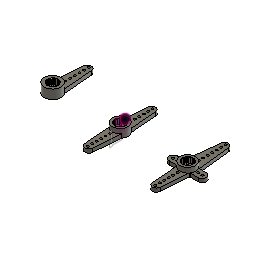
MG90_Arm (Autodesk Fusion 360 design; units mm, degrees)
Autodesk Fusion 360 part; units mm, degrees
sketch "Arm01Base" plane through (0, 0, 0) normal (0, 1, 0) x (1, 0, 0)
  circle A0 centre (0, 0) radius 3.7
  circle A1 centre (0, 0) radius 2.7
  line L0 (0, -3.7) -> (0, 17.2) construction
  circle A2 centre (0, 15.45) radius 1.75
  line L1 (-1.7434, 15.6016) -> (-2.9, 2.2978)
  line L2 (1.7434, 15.6016) -> (2.9, 2.2978)
  circle A3 centre (0, 0) radius 1.375
  circle A4 centre (0, 16.05) radius 0.5
  circle A5 centre (0, 13.98) radius 0.5
  circle A6 centre (0, 11.91) radius 0.5
  circle A7 centre (0, 9.84) radius 0.5
  circle A8 centre (0, 7.77) radius 0.5
  circle A9 centre (0, 5.7) radius 0.5
  point P0 (0, 16.55)
  dimension "d2" = 7.4
  dimension "d3" = 1
  dimension "d4" = 20.9
  dimension "d5" = 3.5
  dimension "d6" = 2.9
  dimension "d7" = 2.75
  dimension "d8" = 1
  dimension "d9" = 0.65
  dimension "d12" = 0
  dimension "d13" = -10.35
  constraint coincident A0.centre A1.centre
  constraint coincident A0 L0.start
  constraint vertical L0
  constraint coincident A0.centre L0
  constraint coincident L0 A2.centre
  constraint coincident L0.end A2
  constraint coincident A2 L1.start
  constraint coincident A0 L1.end
  constraint tangent A2 L1
  constraint symmetric L0 L1.start L2.start
  constraint symmetric L0 L1.end L2.end
  constraint concentric A1 A3
  constraint coincident L0 A4.centre
  constraint coincident A4 P0
  constraint coincident L0 P0
  measures "d2" diameter of A0
  measures "d3" distance of A0 A1
  measures "d4" distance of L0.start L0.end
  measures "d5" diameter of A2
  measures "d6" distance of L0 L1.end
  measures "d7" diameter of A3
  measures "d8" diameter of A4
  measures "d9" distance of L0.end P0
extrude "Extrude1" add sketch "Arm01Base" along normal blind 1.75 contours A0 | A0 A2 L1 L2 A5 | A2 A5 picked at (0.7406, 14.9094) makes body 1
extrude "Extrude2" add sketch "Arm01Base" along normal blind 4.1 contours A0 bodies 1
ref_plane "WorkPlane1" through (0, 1.5, 0) normal (0, 1, 0) x (0, 0, 1)
extrude "Extrude3" add sketch "Arm01Base" against normal blind 0.5 from surface at 1.5 contours A1 bodies 1
sketch "Teeth01" plane through (0, 1.5, 0) normal (0, 1, 0) x (1, 0, 0)
  circle A0 centre (0, 0) radius 2.1 construction
  circle A1 centre (0, 0) radius 2.4 construction
  line L0 (0, 0) -> (0, 2.4) construction
  line L1 (-0.35, 2.3743) -> (0, 2.1)
  line L2 (0.35, 2.3743) -> (0, 2.1)
  line L3 (-1.0666, 2.15) -> (-0.6489, 1.9972)
  line L4 (-0.4008, 2.3663) -> (-0.6489, 1.9972)
  line L5 (-1.6788, 1.7152) -> (-1.2343, 1.6989)
  line L6 (-1.1124, 2.1266) -> (-1.2343, 1.6989)
  line L7 (-2.1266, 1.1124) -> (-1.6989, 1.2343)
  line L8 (-1.7152, 1.6788) -> (-1.6989, 1.2343)
  line L9 (-2.3663, 0.4008) -> (-1.9972, 0.6489)
  line L10 (-2.15, 1.0666) -> (-1.9972, 0.6489)
  line L11 (-2.3743, -0.35) -> (-2.1, 0)
  line L12 (-2.3743, 0.35) -> (-2.1, 0)
  line L13 (-2.15, -1.0666) -> (-1.9972, -0.6489)
  line L14 (-2.3663, -0.4008) -> (-1.9972, -0.6489)
  line L15 (-1.7152, -1.6788) -> (-1.6989, -1.2343)
  line L16 (-2.1266, -1.1124) -> (-1.6989, -1.2343)
  line L17 (-1.1124, -2.1266) -> (-1.2343, -1.6989)
  line L18 (-1.6788, -1.7152) -> (-1.2343, -1.6989)
  line L19 (-0.4008, -2.3663) -> (-0.6489, -1.9972)
  line L20 (-1.0666, -2.15) -> (-0.6489, -1.9972)
  line L21 (0.35, -2.3743) -> (0, -2.1)
  line L22 (-0.35, -2.3743) -> (0, -2.1)
  line L23 (1.0666, -2.15) -> (0.6489, -1.9972)
  line L24 (0.4008, -2.3663) -> (0.6489, -1.9972)
  line L25 (1.6788, -1.7152) -> (1.2343, -1.6989)
  line L26 (1.1124, -2.1266) -> (1.2343, -1.6989)
  line L27 (2.1266, -1.1124) -> (1.6989, -1.2343)
  line L28 (1.7152, -1.6788) -> (1.6989, -1.2343)
  line L29 (2.3663, -0.4008) -> (1.9972, -0.6489)
  line L30 (2.15, -1.0666) -> (1.9972, -0.6489)
  line L31 (2.3743, 0.35) -> (2.1, 0)
  line L32 (2.3743, -0.35) -> (2.1, 0)
  line L33 (2.15, 1.0666) -> (1.9972, 0.6489)
  line L34 (2.3663, 0.4008) -> (1.9972, 0.6489)
  line L35 (1.7152, 1.6788) -> (1.6989, 1.2343)
  line L36 (2.1266, 1.1124) -> (1.6989, 1.2343)
  line L37 (1.1124, 2.1266) -> (1.2343, 1.6989)
  line L38 (1.6788, 1.7152) -> (1.2343, 1.6989)
  line L39 (0.4008, 2.3663) -> (0.6489, 1.9972)
  line L40 (1.0666, 2.15) -> (0.6489, 1.9972)
  circle A2 centre (0, 0) radius 2.7
  circle A3 centre (0, 0) radius 2.4
  dimension "d22" = 4.2
  dimension "d23" = 4.8
  dimension "d24" = 0.35
  dimension "d26" = 360
  constraint coincident A0.centre A1.centre
  constraint concentric A0 A1
  constraint coincident A1 L0.end
  constraint vertical L0
  constraint coincident A1 L1.start
  constraint coincident A0 L1.end
  constraint coincident L0 L1.end
  constraint coincident A1 L2.start
  constraint symmetric L0 L1.start L2.start
  constraint coincident L39.start A3
  measures "d22" diameter of A0
  measures "d23" diameter of A1
  measures "d24" horizontal distance of L0.end L2.start
extrude "Extrude4" add sketch "Teeth01" along normal up to surface (2.6 mm away) contours L1 L2 A3 | L3 L4 A3 | L39 L40 A3 | L5 L6 A3 | L37 L38 A3 | L7 L8 A3 | L35 L36 A3 | L9 L10 A3 | L33 L34 A3 | L11 L12 A3 | L31 L32 A3 | L13 L14 A3 | L29 L30 A3 | L15 L16 A3 | L27 L28 A3 | L17 L18 A3 | L25 L26 A3 | L19 L20 A3 | L23 L24 A3 | L21 L22 A3 | A2 bodies 1
sketch "TeethChamfer01" plane through (0, 0, 0) normal (1, 0, 0) x (0, 0, -1)
  line L0 (3.7, 4.1) -> (-3.7, 4.1) construction
  line L1 (0, 0) -> (0, 4.1) construction
  line L2 (2.3743, 4.1) -> (2.1, 3.8)
  line L3 (2.1, 3.8) -> (2.1, 4.1)
  line L4 (2.3743, 4.1) -> (2.1, 4.1)
  point P0 (2.3743, 4.1)
  point P1 (2.1, 4.1)
  dimension "d29" = 0.3
  constraint coincident L1.start origin
  constraint midpoint L0 L1.end
  constraint coincident P0 L2.start
  constraint coincident L0 P1
  constraint perpendicular L0 L3
  constraint coincident P1 L3.end
  measures "d29" distance of L2.end P1
revolve "Revolve1" cut sketch "TeethChamfer01" angle 360 about axis through (0, 0, 0) along (0, 1, 0) bodies 1
copy_body "Body->Comp1" bodies 1 removing the originals makes body 2 in component "Arm01"
sketch "Arm02Base" plane through (0, 0, 0) normal (0, 1, 0) x (1, 0, 0)
  line L0 (0, 0) -> (30, 0) construction
  circle A0 centre (30, 0) radius 3.45
  circle A1 centre (30, 0) radius 2.25
  line L1 (30, -15.675) -> (30, 15.675) construction
  circle A2 centre (30, 13.925) radius 1.75
  line L2 (28.2556, 14.0649) -> (27.3, 2.1477)
  line L3 (31.7444, 14.0649) -> (32.7, 2.1477)
  circle A3 centre (30, 14.375) radius 0.5
  circle A4 centre (30, 12.405) radius 0.5
  circle A5 centre (30, 10.435) radius 0.5
  circle A6 centre (30, 8.465) radius 0.5
  circle A7 centre (30, 6.495) radius 0.5
  circle A8 centre (30, 4.525) radius 0.5
  line L4 (31.7444, -14.0649) -> (32.7, -2.1477)
  circle A9 centre (30, -13.925) radius 1.75
  circle A10 centre (30, -12.405) radius 0.5
  circle A11 centre (30, -10.435) radius 0.5
  circle A12 centre (30, -8.465) radius 0.5
  circle A13 centre (30, -6.495) radius 0.5
  circle A14 centre (30, -4.525) radius 0.5
  line L5 (28.2556, -14.0649) -> (27.3, -2.1477)
  circle A15 centre (30, -14.375) radius 0.5
  circle A16 centre (30, 0) radius 1.25
  point P0 (30, 14.875)
  dimension "d31" = 30
  dimension "d32" = 6.9
  dimension "d33" = 1.2
  dimension "d34" = 31.35
  dimension "d35" = 3.5
  dimension "d36" = 2.7
  dimension "d37" = 1
  dimension "d38" = 0.8
  dimension "d41" = 0
  dimension "d42" = -9.85
  dimension "d47" = 2.5
  constraint coincident L0.start origin
  constraint horizontal L0
  constraint coincident L0.end A0.centre
  constraint concentric A0 A1
  constraint perpendicular L0 L1
  constraint coincident L1 A2.centre
  constraint coincident L1.end A2
  constraint midpoint L0.end L1
  constraint coincident A2 L2.start
  constraint coincident A0 L2.end
  constraint tangent A2 L2
  constraint symmetric L1 L2.start L3.start
  constraint symmetric L1 L2.end L3.end
  constraint coincident L1 A3.centre
  constraint coincident A3 P0
  constraint coincident L1 P0
  constraint symmetric L0 A2 A9
  constraint symmetric L0 L2.start L5.start
  constraint symmetric L0 L2.end L5.end
  constraint symmetric L0 L3.start L4.start
  constraint symmetric L0 L3.end L4.end
  constraint symmetric L0 A4 A10
  constraint symmetric L0 A5 A11
  constraint symmetric L0 A6 A12
  constraint symmetric L0 A7 A13
  constraint symmetric L0 A8 A14
  constraint symmetric L0 A3 A15
  constraint concentric A0 A16
  measures "d31" distance of L0.start L0.end
  measures "d32" diameter of A0
  measures "d33" distance of A0 A1
  measures "d34" distance of L1.start L1.end
  measures "d35" diameter of A2
  measures "d36" distance of L1 L2.end
  measures "d37" diameter of A3
  measures "d38" distance of L1.end P0
  measures "d47" diameter of A16
extrude "Extrude5" add sketch "Arm02Base" along normal blind 1.65 separate body contours A0 | A0 A2 L2 L3 A4 | A0 L4 A9 A10 L5 | A2 A4 | A9 A10 picked at (30.7004, 13.2473) picked at (30.7004, -13.2473) makes body 3
extrude "Extrude6" add sketch "Arm02Base" along normal blind 3.7 contours A0 bodies 3
ref_plane "WorkPlane2" through (30, 1.45, -8.9113) normal (0, 1, 0) x (1, 0, 0)
extrude "Extrude7" add sketch "Arm02Base" against normal blind 0.5 from surface at 1.45 contours A1 bodies 3
sketch "Teeth02" plane through (0, 1.45, 0) normal (0, 1, 0) x (-1, 0, 0)
  circle A0 centre (-30, 0) radius 1.25
  circle A1 centre (-30, 0) radius 2.25
  line L0 (1.9972, 0.6489) -> (2.15, 1.0666)
  arc A2 (2.15, 1.0666) -> (2.1266, 1.1124) centre (0, 0) ccw
  line L1 (2.1266, 1.1124) -> (1.6989, 1.2343)
  line L2 (1.6989, 1.2343) -> (1.7152, 1.6788)
  arc A3 (1.7152, 1.6788) -> (1.6788, 1.7152) centre (0, 0) ccw
  line L3 (1.6788, 1.7152) -> (1.2343, 1.6989)
  line L4 (1.2343, 1.6989) -> (1.1124, 2.1266)
  arc A4 (1.1124, 2.1266) -> (1.0666, 2.15) centre (0, 0) ccw
  line L5 (1.0666, 2.15) -> (0.6489, 1.9972)
  line L6 (0.6489, 1.9972) -> (0.4008, 2.3663)
  arc A5 (0.4008, 2.3663) -> (0.35, 2.3743) centre (0, 0) ccw
  line L7 (0.35, 2.3743) -> (0, 2.1)
  line L8 (0, 2.1) -> (-0.35, 2.3743)
  arc A6 (-0.35, 2.3743) -> (-0.4008, 2.3663) centre (0, 0) ccw
  line L9 (-0.4008, 2.3663) -> (-0.6489, 1.9972)
  line L10 (-0.6489, 1.9972) -> (-1.0666, 2.15)
  arc A7 (-1.0666, 2.15) -> (-1.1124, 2.1266) centre (0, 0) ccw
  line L11 (-1.1124, 2.1266) -> (-1.2343, 1.6989)
  line L12 (-1.2343, 1.6989) -> (-1.6788, 1.7152)
  arc A8 (-1.6788, 1.7152) -> (-1.7152, 1.6788) centre (0, 0) ccw
  line L13 (-1.7152, 1.6788) -> (-1.6989, 1.2343)
  line L14 (-1.6989, 1.2343) -> (-2.1266, 1.1124)
  arc A9 (-2.1266, 1.1124) -> (-2.15, 1.0666) centre (0, 0) ccw
  line L15 (-2.15, 1.0666) -> (-1.9972, 0.6489)
  line L16 (-1.9972, 0.6489) -> (-2.3663, 0.4008)
  arc A10 (-2.3663, 0.4008) -> (-2.3743, 0.35) centre (0, 0) ccw
  line L17 (-2.3743, 0.35) -> (-2.1, 0)
  line L18 (-2.1, 0) -> (-2.3743, -0.35)
  arc A11 (-2.3743, -0.35) -> (-2.3663, -0.4008) centre (0, 0) ccw
  line L19 (-2.3663, -0.4008) -> (-1.9972, -0.6489)
  line L20 (-1.9972, -0.6489) -> (-2.15, -1.0666)
  arc A12 (-2.15, -1.0666) -> (-2.1266, -1.1124) centre (0, 0) ccw
  line L21 (-2.1266, -1.1124) -> (-1.6989, -1.2343)
  line L22 (-1.6989, -1.2343) -> (-1.7152, -1.6788)
  arc A13 (-1.7152, -1.6788) -> (-1.6788, -1.7152) centre (0, 0) ccw
  line L23 (-1.6788, -1.7152) -> (-1.2343, -1.6989)
  line L24 (-1.2343, -1.6989) -> (-1.1124, -2.1266)
  arc A14 (-1.1124, -2.1266) -> (-1.0666, -2.15) centre (0, 0) ccw
  line L25 (-1.0666, -2.15) -> (-0.6489, -1.9972)
  line L26 (-0.6489, -1.9972) -> (-0.4008, -2.3663)
  arc A15 (-0.4008, -2.3663) -> (-0.35, -2.3743) centre (0, 0) ccw
  line L27 (-0.35, -2.3743) -> (0, -2.1)
  line L28 (0, -2.1) -> (0.35, -2.3743)
  arc A16 (0.35, -2.3743) -> (0.4008, -2.3663) centre (0, 0) ccw
  line L29 (0.4008, -2.3663) -> (0.6489, -1.9972)
  line L30 (0.6489, -1.9972) -> (1.0666, -2.15)
  arc A17 (1.0666, -2.15) -> (1.1124, -2.1266) centre (0, 0) ccw
  line L31 (1.1124, -2.1266) -> (1.2343, -1.6989)
  line L32 (1.2343, -1.6989) -> (1.6788, -1.7152)
  arc A18 (1.6788, -1.7152) -> (1.7152, -1.6788) centre (0, 0) ccw
  line L33 (1.7152, -1.6788) -> (1.6989, -1.2343)
  line L34 (1.6989, -1.2343) -> (2.1266, -1.1124)
  arc A19 (2.1266, -1.1124) -> (2.15, -1.0666) centre (0, 0) ccw
  line L35 (2.15, -1.0666) -> (1.9972, -0.6489)
  line L36 (1.9972, -0.6489) -> (2.3663, -0.4008)
  arc A20 (2.3663, -0.4008) -> (2.3743, -0.35) centre (0, 0) ccw
  line L37 (2.3743, -0.35) -> (2.1, 0)
  line L38 (2.1, 0) -> (2.3743, 0.35)
  arc A21 (2.3743, 0.35) -> (2.3663, 0.4008) centre (0, 0) ccw
  line L39 (2.3663, 0.4008) -> (1.9972, 0.6489)
  circle A22 centre (0, 0) radius 1.375
  arc A23 (-31.7152, -1.6788) -> (-31.6788, -1.7152) centre (-30, 0) ccw
  line L40 (-31.6788, -1.7152) -> (-31.2343, -1.6989)
  line L41 (-31.2343, -1.6989) -> (-31.1124, -2.1266)
  arc A24 (-31.1124, -2.1266) -> (-31.0666, -2.15) centre (-30, 0) ccw
  line L42 (-31.0666, -2.15) -> (-30.6489, -1.9972)
  line L43 (-30.6489, -1.9972) -> (-30.4008, -2.3663)
  arc A25 (-30.4008, -2.3663) -> (-30.35, -2.3743) centre (-30, 0) ccw
  line L44 (-30.35, -2.3743) -> (-30, -2.1)
  line L45 (-30, -2.1) -> (-29.65, -2.3743)
  arc A26 (-29.65, -2.3743) -> (-29.5992, -2.3663) centre (-30, 0) ccw
  line L46 (-29.5992, -2.3663) -> (-29.3511, -1.9972)
  line L47 (-29.3511, -1.9972) -> (-28.9334, -2.15)
  arc A27 (-28.9334, -2.15) -> (-28.8876, -2.1266) centre (-30, 0) ccw
  line L48 (-28.8876, -2.1266) -> (-28.7657, -1.6989)
  line L49 (-28.7657, -1.6989) -> (-28.3212, -1.7152)
  arc A28 (-28.3212, -1.7152) -> (-28.2848, -1.6788) centre (-30, 0) ccw
  line L50 (-28.2848, -1.6788) -> (-28.3011, -1.2343)
  line L51 (-28.3011, -1.2343) -> (-27.8734, -1.1124)
  arc A29 (-27.8734, -1.1124) -> (-27.85, -1.0666) centre (-30, 0) ccw
  line L52 (-27.85, -1.0666) -> (-28.0028, -0.6489)
  line L53 (-28.0028, -0.6489) -> (-27.6337, -0.4008)
  arc A30 (-27.6337, -0.4008) -> (-27.6257, -0.35) centre (-30, 0) ccw
  line L54 (-27.6257, -0.35) -> (-27.9, 0)
  line L55 (-27.9, 0) -> (-27.6257, 0.35)
  arc A31 (-27.6257, 0.35) -> (-27.6337, 0.4008) centre (-30, 0) ccw
  line L56 (-27.6337, 0.4008) -> (-28.0028, 0.6489)
  line L57 (-28.0028, 0.6489) -> (-27.85, 1.0666)
  arc A32 (-27.85, 1.0666) -> (-27.8734, 1.1124) centre (-30, 0) ccw
  line L58 (-27.8734, 1.1124) -> (-28.3011, 1.2343)
  line L59 (-28.3011, 1.2343) -> (-28.2848, 1.6788)
  arc A33 (-28.2848, 1.6788) -> (-28.3212, 1.7152) centre (-30, 0) ccw
  line L60 (-28.3212, 1.7152) -> (-28.7657, 1.6989)
  line L61 (-28.7657, 1.6989) -> (-28.8876, 2.1266)
  arc A34 (-28.8876, 2.1266) -> (-28.9334, 2.15) centre (-30, 0) ccw
  line L62 (-28.9334, 2.15) -> (-29.3511, 1.9972)
  line L63 (-29.3511, 1.9972) -> (-29.5992, 2.3663)
  arc A35 (-29.5992, 2.3663) -> (-29.65, 2.3743) centre (-30, 0) ccw
  line L64 (-29.65, 2.3743) -> (-30, 2.1)
  line L65 (-30, 2.1) -> (-30.35, 2.3743)
  arc A36 (-30.35, 2.3743) -> (-30.4008, 2.3663) centre (-30, 0) ccw
  line L66 (-30.4008, 2.3663) -> (-30.6489, 1.9972)
  line L67 (-30.6489, 1.9972) -> (-31.0666, 2.15)
  arc A37 (-31.0666, 2.15) -> (-31.1124, 2.1266) centre (-30, 0) ccw
  line L68 (-31.1124, 2.1266) -> (-31.2343, 1.6989)
  line L69 (-31.2343, 1.6989) -> (-31.6788, 1.7152)
  arc A38 (-31.6788, 1.7152) -> (-31.7152, 1.6788) centre (-30, 0) ccw
  line L70 (-31.7152, 1.6788) -> (-31.6989, 1.2343)
  line L71 (-31.6989, 1.2343) -> (-32.1266, 1.1124)
  arc A39 (-32.1266, 1.1124) -> (-32.15, 1.0666) centre (-30, 0) ccw
  line L72 (-32.15, 1.0666) -> (-31.9972, 0.6489)
  line L73 (-31.9972, 0.6489) -> (-32.3663, 0.4008)
  arc A40 (-32.3663, 0.4008) -> (-32.3743, 0.35) centre (-30, 0) ccw
  line L74 (-32.3743, 0.35) -> (-32.1, 0)
  line L75 (-32.1, 0) -> (-32.3743, -0.35)
  arc A41 (-32.3743, -0.35) -> (-32.3663, -0.4008) centre (-30, 0) ccw
  line L76 (-32.3663, -0.4008) -> (-31.9972, -0.6489)
  line L77 (-31.9972, -0.6489) -> (-32.15, -1.0666)
  arc A42 (-32.15, -1.0666) -> (-32.1266, -1.1124) centre (-30, 0) ccw
  line L78 (-32.1266, -1.1124) -> (-31.6989, -1.2343)
  line L79 (-31.6989, -1.2343) -> (-31.7152, -1.6788)
  circle A43 centre (-30, 0) radius 2.4
  dimension "d54" = -30
  dimension "d55" = 0
  constraint concentric A0 A43
  constraint coincident L41.end A43
extrude "Extrude8" cut sketch "Teeth02" along normal up to surface (2.25 mm away) contours A1 L55 A31 L56 A43 | A1 L53 A30 L54 A43 | A1 L57 A32 L58 A43 | A1 L51 A29 L52 A43 | A1 L59 A33 L60 A43 | A1 L49 A28 L50 A43 | A1 L61 A34 L62 A43 | A1 L47 A27 L48 A43 | A1 L63 A35 L64 A43 | A1 L45 A26 L46 A43 | A1 L65 A36 L66 A43 | A1 L43 A25 L44 A43 | A1 L67 A37 L68 A43 | A1 L41 A24 L42 A43 | A1 L69 A38 L70 A43 | A1 A23 L40 L79 A43 | A1 L71 A39 L72 A43 | A1 L77 A42 L78 A43 | A1 L73 A40 L74 A43 | A1 L75 A41 L76 A43 bodies 3
extrude "Extrude9" add sketch "Teeth02" along normal up to surface (2.25 mm away) contours A1 L54 L55 | A1 L56 L57 | A1 L52 L53 | A1 L58 L59 | A1 L50 L51 | A1 L60 L61 | A1 L48 L49 | A1 L62 L63 | A1 L46 L47 | A1 L64 L65 | A1 L44 L45 | A1 L66 L67 | A1 L42 L43 | A1 L68 L69 | A1 L40 L41 | A1 L70 L71 | A1 L78 L79 | A1 L72 L73 | A1 L76 L77 | A1 L74 L75 bodies 3
ref_plane "WorkPlane3" through (30, 0, 0) normal (1, 0, 0) x (0, 1, 0)
sketch "TeethChamfer02" plane through (30, 0, 0) normal (1, 0, 0) x (0, 0, -1)
  line L0 (2.1, 3.8) -> (2.1, 4.1) construction
  line L1 (2.3743, 4.1) -> (2.1, 4.1) construction
  line L2 (2.3743, 4.1) -> (2.1, 3.8) construction
  line L3 (0, 0) -> (0, 4.1) construction
  line L4 (2.1, 3.7) -> (2.3743, 3.7)
  line L5 (2.3743, 3.7) -> (2.3743, 4.1) construction
  line L6 (2.3743, 3.7) -> (2.1, 3.4)
  line L7 (2.1, 1.45) -> (2.1, 3.7)
  point P0 (2.1, 3.7)
  constraint parallel L1 L4
  constraint coincident L1.start L2.start
  constraint perpendicular L1 L5
  constraint coincident P0 L4.start
  constraint parallel L2 L6
  constraint coincident L6.end L7
revolve "Revolve3" cut sketch "TeethChamfer02" angle 360 about axis through (30, 0, 0) along (0, 1, 0) bodies 3
copy_body "Body->Comp2" bodies 3 removing the originals makes body 4 in component "Arm02"
sketch "Arm03Base" plane through (0, 0, 0) normal (0, 1, 0) x (1, 0, 0)
  line L0 (0, 0) -> (60, 0) construction
  circle A0 centre (60, 0) radius 3.45
  circle A1 centre (60, 0) radius 1.25
  circle A2 centre (60, 0) radius 2.25
  arc A3 (27.3, -2.1477) -> (32.7, -2.1477) centre (30, 0) ccw construction
  line L1 (27.3, -2.1477) -> (28.2556, -14.0649)
  arc A4 (28.2556, -14.0649) -> (31.7444, -14.0649) centre (30, -13.925) ccw
  line L2 (31.7444, -14.0649) -> (32.7, -2.1477)
  circle A5 centre (30, -4.525) radius 0.5
  circle A6 centre (30, -6.495) radius 0.5
  circle A7 centre (30, -8.465) radius 0.5
  circle A8 centre (30, -10.435) radius 0.5
  circle A9 centre (30, -12.405) radius 0.5
  circle A10 centre (30, -14.375) radius 0.5
  arc A11 (32.7, 2.1477) -> (27.3, 2.1477) centre (30, 0) ccw construction
  line L3 (32.7, 2.1477) -> (31.7444, 14.0649) construction
  arc A12 (31.7444, 14.0649) -> (28.2556, 14.0649) centre (30, 13.925) ccw construction
  line L4 (28.2556, 14.0649) -> (27.3, 2.1477) construction
  circle A13 centre (30, 12.405) radius 0.5
  circle A14 centre (30, 6.495) radius 0.5
  circle A15 centre (30, 4.525) radius 0.5
  circle A16 centre (30, 14.375) radius 0.5
  circle A17 centre (30, 10.435) radius 0.5
  circle A18 centre (30, 8.465) radius 0.5
  arc A19 (58.2556, -14.0649) -> (61.7444, -14.0649) centre (60, -13.925) ccw
  line L5 (61.7444, -14.0649) -> (62.7, -2.1477)
  circle A20 centre (60, -10.435) radius 0.5
  circle A21 centre (60, -12.405) radius 0.5
  circle A22 centre (60, -14.375) radius 0.5
  circle A23 centre (60, -8.465) radius 0.5
  circle A24 centre (60, -6.495) radius 0.5
  line L6 (57.3, -2.1477) -> (58.2556, -14.0649)
  circle A25 centre (60, -4.525) radius 0.5
  line L7 (60, -15.675) -> (60, 18.025) construction
  circle A26 centre (60, 16.825) radius 0.5
  circle A27 centre (60, 14.8167) radius 0.5
  circle A28 centre (60, 12.8083) radius 0.5
  circle A29 centre (60, 10.8) radius 0.5
  circle A30 centre (60, 8.7917) radius 0.5
  circle A31 centre (60, 6.7833) radius 0.5
  circle A32 centre (60, 4.775) radius 0.5
  circle A33 centre (60, 16.275) radius 1.75
  line L8 (58.2599, 16.4608) -> (56.7, 1.85)
  circle A34 centre (53.45, 0) radius 0.5
  circle A35 centre (53.6, 0) radius 1.85
  line L9 (53.6, 1.85) -> (57.088, 1.85)
  line L10 (53.6, 0) -> (53.6, 1.85) construction
  line L11 (53.6, -1.85) -> (57.088, -1.85)
  circle A36 centre (55.4, 0) radius 0.5
  line L12 (66.4, 1.85) -> (62.912, 1.85)
  circle A37 centre (66.4, 0) radius 1.85
  circle A38 centre (66.55, 0) radius 0.5
  circle A39 centre (64.6, 0) radius 0.5
  line L13 (66.4, -1.85) -> (62.912, -1.85)
  line L14 (61.7401, 16.4608) -> (63.3, 1.85)
  point P0 (60, 17.325)
  point P1 (51.75, 0)
  point P2 (52.95, 0)
  point P3 (55.9, 0)
  point P4 (57.75, 0)
  dimension "d62" = 60
  dimension "d63" = 6.9
  dimension "d64" = 2.5
  dimension "d65" = 1.2
  dimension "d79" = 30
  dimension "d80" = 0
  dimension "d81" = 1
  dimension "d84" = 0
  dimension "d85" = -12.05
  dimension "d86" = 33.7
  dimension "d87" = 0.7
  dimension "d88" = 3.5
  dimension "d89" = 3.3
  dimension "d90" = 1
  dimension "d91" = 3.7
  dimension "d92" = 8.25
  dimension "d93" = 1.2
  dimension "d94" = 1
  dimension "d95" = 1.95
  dimension "d96" = 1.85
  constraint coincident L0.start origin
  constraint horizontal L0
  constraint coincident L0.end A0.centre
  constraint concentric A0 A1
  constraint concentric A0 A2
  constraint midpoint A19 L7.start
  constraint vertical L7
  constraint coincident L7 A26.centre
  constraint coincident A26 P0
  constraint coincident L7 P0
  constraint coincident L7 A33.centre
  constraint coincident L7.end A33
  constraint coincident A33 L8.start
  constraint tangent A33 L8
  constraint coincident L0 A34.centre
  constraint coincident L0 A35.centre
  constraint coincident A35 L9.start
  constraint coincident A0 L9.end
  constraint horizontal L9
  constraint coincident L8.end L9
  constraint coincident A35 P1
  constraint coincident L0 P1
  constraint coincident A34 P2
  constraint coincident L0 P2
  constraint coincident A35.centre L10.start
  constraint vertical L10
  constraint symmetric L0 L9.start L11.start
  constraint symmetric L0 L9.end L11.end
  constraint coincident L0 A36.centre
  constraint coincident A36 P3
  constraint coincident L0 P3
  constraint coincident A2 P4
  constraint coincident L0 P4
  constraint symmetric L7 L8.start L14.start
  constraint symmetric L7 L8.end L14.end
  constraint symmetric L7 A34 A38
  constraint symmetric L7 A35 A37
  constraint symmetric L7 L9.start L12.start
  constraint symmetric L7 L9.end L12.end
  constraint symmetric L7 L11.start L13.start
  constraint symmetric L7 L11.end L13.end
  constraint symmetric L7 A36 A39
  measures "d62" distance of L0.start L0.end
  measures "d63" diameter of A0
  measures "d64" diameter of A1
  measures "d65" distance of A0 A2
  measures "d81" diameter of A26
  measures "d86" distance of L7.start L7.end
  measures "d87" distance of L7.end P0
  measures "d88" diameter of A33
  measures "d89" distance of L7 L8.end
  measures "d90" diameter of A34
  measures "d91" diameter of A35
  measures "d92" distance of L0.end P1
  measures "d93" distance of P1 P2
  measures "d94" diameter of A36
  measures "d95" distance of A34.centre A36.centre
  measures "d96" distance of P3 P4
extrude "Extrude10" add sketch "Arm03Base" along normal blind 1.6 separate body contours A0 | A0 L12 A37 A39 L13 | A0 A27 A33 L8 L9 L12 L14 | A0 A35 L9 L11 A36 | A0 A19 L5 L6 | A37 A39 | A27 A33 | A35 A36 picked at (65.3708, 0.6009) picked at (60.7393, 15.7217) picked at (54.625, -0.5957) makes body 5
extrude "Extrude11" add sketch "Arm03Base" along normal blind 3.8 contours A0 bodies 5
extrude "Extrude12" add sketch "Arm03Base" along normal up to surface (0.5 mm away) from surface at 0.95 contours A2 bodies 5
sketch "Teeth03" plane through (0, 1.45, 0) normal (0, 1, 0) x (-1, 0, 0)
  circle A0 centre (-60, 0) radius 1.25
  circle A1 centre (-60, 0) radius 2.25
  line L0 (-31.0666, -2.15) -> (-30.6489, -1.9972)
  line L1 (-30.6489, -1.9972) -> (-30.4008, -2.3663)
  arc A2 (-30.4008, -2.3663) -> (-30.35, -2.3743) centre (-30, 0) ccw
  line L2 (-30.35, -2.3743) -> (-30, -2.1)
  line L3 (-30, -2.1) -> (-29.65, -2.3743)
  arc A3 (-29.65, -2.3743) -> (-29.5992, -2.3663) centre (-30, 0) ccw
  line L4 (-29.5992, -2.3663) -> (-29.3511, -1.9972)
  line L5 (-29.3511, -1.9972) -> (-28.9334, -2.15)
  arc A4 (-28.9334, -2.15) -> (-28.8876, -2.1266) centre (-30, 0) ccw
  line L6 (-28.8876, -2.1266) -> (-28.7657, -1.6989)
  line L7 (-28.7657, -1.6989) -> (-28.3212, -1.7152)
  arc A5 (-28.3212, -1.7152) -> (-28.2848, -1.6788) centre (-30, 0) ccw
  line L8 (-28.2848, -1.6788) -> (-28.3011, -1.2343)
  line L9 (-28.3011, -1.2343) -> (-27.8734, -1.1124)
  arc A6 (-27.8734, -1.1124) -> (-27.85, -1.0666) centre (-30, 0) ccw
  line L10 (-27.85, -1.0666) -> (-28.0028, -0.6489)
  line L11 (-28.0028, -0.6489) -> (-27.6337, -0.4008)
  arc A7 (-27.6337, -0.4008) -> (-27.6257, -0.35) centre (-30, 0) ccw
  line L12 (-27.6257, -0.35) -> (-27.9, 0)
  line L13 (-27.9, 0) -> (-27.6257, 0.35)
  arc A8 (-27.6257, 0.35) -> (-27.6337, 0.4008) centre (-30, 0) ccw
  line L14 (-27.6337, 0.4008) -> (-28.0028, 0.6489)
  line L15 (-28.0028, 0.6489) -> (-27.85, 1.0666)
  arc A9 (-27.85, 1.0666) -> (-27.8734, 1.1124) centre (-30, 0) ccw
  line L16 (-27.8734, 1.1124) -> (-28.3011, 1.2343)
  line L17 (-28.3011, 1.2343) -> (-28.2848, 1.6788)
  arc A10 (-28.2848, 1.6788) -> (-28.3212, 1.7152) centre (-30, 0) ccw
  line L18 (-28.3212, 1.7152) -> (-28.7657, 1.6989)
  line L19 (-28.7657, 1.6989) -> (-28.8876, 2.1266)
  arc A11 (-28.8876, 2.1266) -> (-28.9334, 2.15) centre (-30, 0) ccw
  line L20 (-28.9334, 2.15) -> (-29.3511, 1.9972)
  line L21 (-29.3511, 1.9972) -> (-29.5992, 2.3663)
  arc A12 (-29.5992, 2.3663) -> (-29.65, 2.3743) centre (-30, 0) ccw
  line L22 (-29.65, 2.3743) -> (-30, 2.1)
  line L23 (-30, 2.1) -> (-30.35, 2.3743)
  arc A13 (-30.35, 2.3743) -> (-30.4008, 2.3663) centre (-30, 0) ccw
  line L24 (-30.4008, 2.3663) -> (-30.6489, 1.9972)
  line L25 (-30.6489, 1.9972) -> (-31.0666, 2.15)
  arc A14 (-31.0666, 2.15) -> (-31.1124, 2.1266) centre (-30, 0) ccw
  line L26 (-31.1124, 2.1266) -> (-31.2343, 1.6989)
  line L27 (-31.2343, 1.6989) -> (-31.6788, 1.7152)
  arc A15 (-31.6788, 1.7152) -> (-31.7152, 1.6788) centre (-30, 0) ccw
  line L28 (-31.7152, 1.6788) -> (-31.6989, 1.2343)
  line L29 (-31.6989, 1.2343) -> (-32.1266, 1.1124)
  arc A16 (-32.1266, 1.1124) -> (-32.15, 1.0666) centre (-30, 0) ccw
  line L30 (-32.15, 1.0666) -> (-31.9972, 0.6489)
  line L31 (-31.9972, 0.6489) -> (-32.3663, 0.4008)
  arc A17 (-32.3663, 0.4008) -> (-32.3743, 0.35) centre (-30, 0) ccw
  line L32 (-32.3743, 0.35) -> (-32.1, 0)
  line L33 (-32.1, 0) -> (-32.3743, -0.35)
  arc A18 (-32.3743, -0.35) -> (-32.3663, -0.4008) centre (-30, 0) ccw
  line L34 (-32.3663, -0.4008) -> (-31.9972, -0.6489)
  line L35 (-31.9972, -0.6489) -> (-32.15, -1.0666)
  arc A19 (-32.15, -1.0666) -> (-32.1266, -1.1124) centre (-30, 0) ccw
  line L36 (-32.1266, -1.1124) -> (-31.6989, -1.2343)
  line L37 (-31.6989, -1.2343) -> (-31.7152, -1.6788)
  arc A20 (-31.7152, -1.6788) -> (-31.6788, -1.7152) centre (-30, 0) ccw
  line L38 (-31.6788, -1.7152) -> (-31.2343, -1.6989)
  line L39 (-31.2343, -1.6989) -> (-31.1124, -2.1266)
  arc A21 (-31.1124, -2.1266) -> (-31.0666, -2.15) centre (-30, 0) ccw
  circle A22 centre (-30, 0) radius 2.4
  line L40 (-60.6489, 1.9972) -> (-61.0666, 2.15)
  line L41 (-61.2343, -1.6989) -> (-61.1124, -2.1266)
  line L42 (-60, 2.1) -> (-60.35, 2.3743)
  line L43 (-58.9334, 2.15) -> (-59.3511, 1.9972)
  line L44 (-61.1124, 2.1266) -> (-61.2343, 1.6989)
  line L45 (-58.3212, 1.7152) -> (-58.7657, 1.6989)
  line L46 (-59.65, 2.3743) -> (-60, 2.1)
  arc A23 (-58.8876, 2.1266) -> (-58.9334, 2.15) centre (-60, 0) ccw
  line L47 (-58.8876, -2.1266) -> (-58.7657, -1.6989)
  line L48 (-58.3011, 1.2343) -> (-58.2848, 1.6788)
  line L49 (-58.7657, 1.6989) -> (-58.8876, 2.1266)
  line L50 (-61.7152, 1.6788) -> (-61.6989, 1.2343)
  line L51 (-57.9, 0) -> (-57.6257, 0.35)
  line L52 (-58.0028, 0.6489) -> (-57.85, 1.0666)
  line L53 (-62.3743, 0.35) -> (-62.1, 0)
  arc A24 (-57.6257, 0.35) -> (-57.6337, 0.4008) centre (-60, 0) ccw
  circle A25 centre (-60, 0) radius 2.4
  arc A26 (-58.2848, 1.6788) -> (-58.3212, 1.7152) centre (-60, 0) ccw
  arc A27 (-59.5992, 2.3663) -> (-59.65, 2.3743) centre (-60, 0) ccw
  line L54 (-57.6257, -0.35) -> (-57.9, 0)
  line L55 (-60, -2.1) -> (-59.65, -2.3743)
  line L56 (-62.1266, -1.1124) -> (-61.6989, -1.2343)
  line L57 (-58.7657, -1.6989) -> (-58.3212, -1.7152)
  line L58 (-60.35, -2.3743) -> (-60, -2.1)
  line L59 (-57.85, -1.0666) -> (-58.0028, -0.6489)
  line L60 (-61.2343, 1.6989) -> (-61.6788, 1.7152)
  line L61 (-57.6337, 0.4008) -> (-58.0028, 0.6489)
  line L62 (-61.9972, -0.6489) -> (-62.15, -1.0666)
  line L63 (-60.6489, -1.9972) -> (-60.4008, -2.3663)
  arc A28 (-61.1124, -2.1266) -> (-61.0666, -2.15) centre (-60, 0) ccw
  line L64 (-62.1, 0) -> (-62.3743, -0.35)
  line L65 (-61.6788, -1.7152) -> (-61.2343, -1.6989)
  arc A29 (-59.65, -2.3743) -> (-59.5992, -2.3663) centre (-60, 0) ccw
  line L66 (-58.0028, -0.6489) -> (-57.6337, -0.4008)
  line L67 (-58.2848, -1.6788) -> (-58.3011, -1.2343)
  line L68 (-61.6989, -1.2343) -> (-61.7152, -1.6788)
  line L69 (-59.3511, 1.9972) -> (-59.5992, 2.3663)
  line L70 (-61.9972, 0.6489) -> (-62.3663, 0.4008)
  arc A30 (-60.35, 2.3743) -> (-60.4008, 2.3663) centre (-60, 0) ccw
  arc A31 (-62.1266, 1.1124) -> (-62.15, 1.0666) centre (-60, 0) ccw
  arc A32 (-61.6788, 1.7152) -> (-61.7152, 1.6788) centre (-60, 0) ccw
  line L71 (-60.4008, 2.3663) -> (-60.6489, 1.9972)
  arc A33 (-62.3663, 0.4008) -> (-62.3743, 0.35) centre (-60, 0) ccw
  arc A34 (-62.3743, -0.35) -> (-62.3663, -0.4008) centre (-60, 0) ccw
  line L72 (-57.8734, 1.1124) -> (-58.3011, 1.2343)
  line L73 (-62.15, 1.0666) -> (-61.9972, 0.6489)
  arc A35 (-61.0666, 2.15) -> (-61.1124, 2.1266) centre (-60, 0) ccw
  line L74 (-58.3011, -1.2343) -> (-57.8734, -1.1124)
  arc A36 (-57.85, 1.0666) -> (-57.8734, 1.1124) centre (-60, 0) ccw
  arc A37 (-61.7152, -1.6788) -> (-61.6788, -1.7152) centre (-60, 0) ccw
  arc A38 (-57.6337, -0.4008) -> (-57.6257, -0.35) centre (-60, 0) ccw
  line L75 (-59.3511, -1.9972) -> (-58.9334, -2.15)
  arc A39 (-58.3212, -1.7152) -> (-58.2848, -1.6788) centre (-60, 0) ccw
  arc A40 (-62.15, -1.0666) -> (-62.1266, -1.1124) centre (-60, 0) ccw
  line L76 (-59.5992, -2.3663) -> (-59.3511, -1.9972)
  line L77 (-61.6989, 1.2343) -> (-62.1266, 1.1124)
  line L78 (-62.3663, -0.4008) -> (-61.9972, -0.6489)
  arc A41 (-57.8734, -1.1124) -> (-57.85, -1.0666) centre (-60, 0) ccw
  arc A42 (-60.4008, -2.3663) -> (-60.35, -2.3743) centre (-60, 0) ccw
  line L79 (-61.0666, -2.15) -> (-60.6489, -1.9972)
  arc A43 (-58.9334, -2.15) -> (-58.8876, -2.1266) centre (-60, 0) ccw
  dimension "d106" = -30
  dimension "d107" = 0
extrude "Extrude13" cut sketch "Teeth03" along normal up to surface (2.35 mm away) contours A1 L51 A24 A25 L61 | A1 A25 L54 L66 A38 | A1 L52 A25 L72 A36 | A1 A25 L59 L74 A41 | A1 L45 L48 A25 A26 | A1 A25 L57 L67 A39 | A1 L43 A23 L49 A25 | A1 L47 A25 L75 A43 | A1 L46 A25 A27 L69 | A1 A25 L55 A29 L76 | A1 L42 A25 A30 L71 | A1 A25 L58 L63 A42 | A1 L40 L44 A25 A35 | A1 L41 A25 A28 L79 | A1 L50 A25 L60 A32 | A1 A25 L65 L68 A37 | A1 A25 A31 L73 L77 | A1 A25 L56 L62 A40 | A1 L53 A25 L70 A33 | A1 A25 L64 A34 L78 bodies 5
extrude "Extrude14" add sketch "Teeth03" along normal up to surface (2.35 mm away) contours A1 L51 L54 | A1 L52 L61 | A1 L59 L66 | A1 L48 L72 | A1 L67 L74 | A1 L45 L49 | A1 L47 L57 | A1 L43 L69 | A1 L75 L76 | A1 L42 L46 | A1 L55 L58 | A1 L40 L71 | A1 L63 L79 | A1 L44 L60 | A1 L41 L65 | A1 L50 L77 | A1 L56 L68 | A1 L70 L73 | A1 L62 L78 | A1 L53 L64 bodies 5
ref_plane "WorkPlane4" through (60, 1.45, -2.1) normal (-1, 0, 0) x (0, -1, 0)
sketch "TeethChamfer03" plane through (60, 1.45, -2.1) normal (-1, 0, 0) x (0, 0, -1)
  line L0 (0, -2.25) -> (0.2743, -2.25) construction
  line L1 (0.2743, -2.25) -> (0, -1.95) construction
  line L2 (0, 0) -> (0, -2.25) construction
  line L3 (-2.1, 1.45) -> (-2.1, -2.65) construction
  line L4 (0, -2.35) -> (0.2743, -2.35)
  line L5 (0.2743, -2.35) -> (0.2743, -2.25)
  line L6 (0.2743, -2.35) -> (0, -2.05)
  line L7 (0, -2.05) -> (0, -2.35)
  point P0 (0, -2.35)
  constraint horizontal L4
  constraint coincident L0.end L1.start
  constraint vertical L5
  constraint coincident P0 L4.start
  constraint coincident L2 L6.end
  constraint parallel L1 L6
revolve "Revolve4" cut sketch "TeethChamfer03" angle 360 about axis through (60, 0, 0) along (0, 1, 0) bodies 5
component "Arm01" placed x (1, 0, 0) y (0, 1, 0) z (0, 0, 1) at (0, 0, 0)
component "Arm02" placed x (1, 0, 0) y (0, 1, 0) z (0, 0, 1) at (0, 0, 0)
equation "SA1_Hull_D = 7.4 mm"
equation "d2 = SA1_Hull_D"
equation "d6 = ( 5.8 / 2 ) * 1 mm"
equation "d36 = ( 5.4 / 2 ) * 1 mm"
named bodies: "Arm01", "Arm02", "Arm03"
